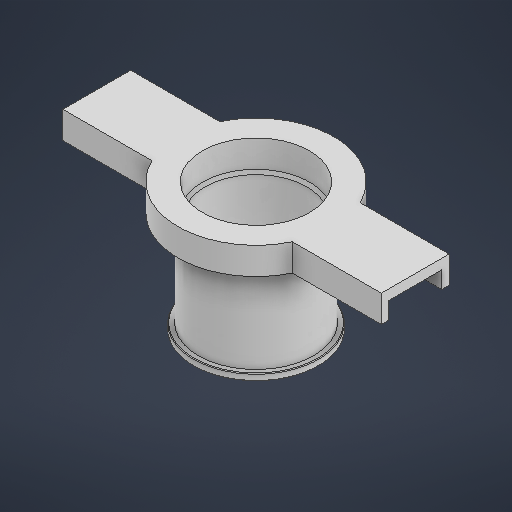
# Autodesk Inventor part: Cylinder  Segment - 11
Saved by Autodesk Inventor 2025 (Build 290162000, 162)
## iProperties
Created: 2024-04-11
Part Number: Cylinder  Segment - 11
Material: Generic
Document SubType Name: Modeling
Designer: Thienan Hoang
Density: 1 g/cm^3
Appearance: Default
Author: Thienan Hoang
Autodesk Inventor part; units mm, degrees
ref_plane "YZ Plane" through (0, 0, 0) normal (1, 0, 0) x (0, 1, 0)
ref_plane "XZ Plane" through (0, 0, 0) normal (0, 1, 0) x (-1, 0, 0)
ref_plane "XY Plane" through (0, 0, 0) normal (0, 0, 1) x (1, 0, 0)
sketch "Sketch1" plane through (0, 0, 0) normal (0, 1, 0) x (-1, 0, 0)
  circle A0 centre (0, 0) radius 46.125
  circle A1 centre (0, 0) radius 42.5
  circle A2 centre (0, 0) radius 37.5
  circle A3 centre (0, 0) radius 9.5
  dimension "Absolute_Diameter" = 92.25
  dimension "Diameter_No_Outer_Lip" = 85
  dimension "Inner_Cylinder_Diameter" = 75
  dimension "Lip_Diameter" = 19
  constraints: 4 centre point, 4 coincident
  measures "Absolute_Diameter" diameter of A0
  measures "Diameter_No_Outer_Lip" diameter of A1
  measures "Inner_Cylinder_Diameter" diameter of A2
  measures "Lip_Diameter" diameter of A3
extrude "Extrusion1" add sketch "Sketch1" along normal blind 5 contours A0
extrude "Extrusion2" add sketch "Sketch1" along normal blind 75 contours A1
sketch "Sketch2" plane through (0, 75, 0) normal (0, 1, 0) x (1, 0, 0)
  circle A0 centre (0, 0) radius 42.5
  circle A1 centre (0, 0) radius 50
  dimension "Lip_Diameter_Out" = 85
  dimension "Inner_Lip_Diameter" = 100
  constraints: 2 centre point, 1 coincident
  measures "Lip_Diameter_Out" diameter of A0
  measures "Inner_Lip_Diameter" diameter of A1
extrude "Extrusion7" [suppressed]
chamfer "Chamfer1" distance 0.5 angle 45 1 edges at (42.5, 75, 0)
chamfer "Chamfer2" distance 0.5 angle 45 3 edges at (46.125, 5, 0) (46.125, 0, 0) (37.5, 0, 0)
sketch "Sketch3" plane through (0, 5, 0) normal (0, 1, 0) x (1, 0, 0)
  circle A0 centre (0, 0) radius 127.5
  circle A1 centre (-127.5, 0) radius 2.5
  circle A2 centre (-103.1497, -74.9426) radius 2.5
  circle A3 centre (-39.3997, -121.2597) radius 2.5
  circle A4 centre (39.3997, -121.2597) radius 2.5
  circle A5 centre (103.1497, -74.9426) radius 2.5
  circle A6 centre (127.5, 0) radius 2.5
  circle A7 centre (103.1497, 74.9426) radius 2.5
  circle A8 centre (39.3997, 121.2597) radius 2.5
  circle A9 centre (-39.3997, 121.2597) radius 2.5
  circle A10 centre (-103.1497, 74.9426) radius 2.5
  dimension "d27" = 255
  dimension "d28" = 5
  dimension "d31" = 360
  constraints: 10 centre point, 1 coincident, 1 horizontal alignment, 23 other
  measures "d28" diameter of A1
extrude "Extrusion8" [suppressed]
chamfer "Chamfer3" distance 2 angle 45 1 edges at (37.5, 75, 0)
sketch "Sketch5" plane through (0, 75, 0) normal (0, 1, 0) x (1, 0, 0)
  circle A0 centre (0, 0) radius 39.5
  circle A1 centre (0, 0) radius 38 projected
  line L0 (117.5, 25) -> (117.5, -25)
  line L1 (-117.5, -25) -> (-117.5, 25)
  line L2 (-117.5, 25) -> (-51.7808, 25)
  line L3 (51.7808, 25) -> (117.5, 25)
  line L4 (117.5, -25) -> (51.7808, -25)
  line L5 (-51.7808, -25) -> (-117.5, -25)
  arc A2 (-51.7808, -25) -> (51.7808, -25) centre (0, 0) ccw
  arc A3 (51.7808, 25) -> (-51.7808, 25) centre (0, 0) ccw
  dimension "d54" = 50
  dimension "d55" = 235
  constraints: 12 end point, 5 parallel, 4 point on circle, 3 centre point, 2 coincident, 2 horizontal, 2 perpendicular
  measures "d54" distance of L0.start L0.end
  measures "d55" distance between parallel lines of L0 L1
extrude "Extrusion9" add sketch "Sketch5" along normal blind 20 contours L0 L4 A2 L5 L1 L2 A3 L3
sketch "Sketch6" plane through (0, 75, 0) normal (0, -1, 0) x (1, 0, 0)
  line L0 (117.25, -22) -> (-117.25, -22)
  line L1 (-117.25, -22) -> (-117.25, 22)
  line L2 (-117.25, 22) -> (117.25, 22)
  line L3 (117.25, 22) -> (117.25, -22)
  line L4 (117.25, -22) -> (-117.25, 22) construction
  line L5 (-117.25, -22) -> (117.25, 22) construction
  line L6 (145.5, -19.625) -> (92, -19.625)
  line L7 (89, -16.625) -> (89, 16.625)
  line L8 (92, 19.625) -> (145.5, 19.625)
  line L9 (145.5, 19.625) -> (145.5, -19.625)
  line L10 (145.5, -19.625) -> (89, 19.625) construction
  line L11 (89, -19.625) -> (145.5, 19.625) construction
  line L12 (-92, -19.625) -> (-145.5, -19.625)
  line L13 (-145.5, -19.625) -> (-145.5, 19.625)
  line L14 (-145.5, 19.625) -> (-92, 19.625)
  line L15 (-89, 16.625) -> (-89, -16.625)
  line L16 (-89, -19.625) -> (-145.5, 19.625) construction
  line L17 (-145.5, -19.625) -> (-89, 19.625) construction
  arc A0 (-92, -19.625) -> (-89, -16.625) centre (-92, -16.625) ccw
  arc A1 (-89, 16.625) -> (-92, 19.625) centre (-92, 16.625) ccw
  arc A2 (89, -16.625) -> (92, -19.625) centre (92, -16.625) ccw
  arc A3 (92, 19.625) -> (89, 16.625) centre (92, 16.625) ccw
  point P0 (0, 0)
  point P1 (117.25, 0)
  point P2 (-117.25, 0)
  dimension "d58" = 234.5
  dimension "d59" = 44
  dimension "d60" = 56.5
  dimension "d61" = 39.25
  dimension "d62" = 56.5
  dimension "d63" = 39.25
  dimension "d64" = 3
  constraints: 36 end point, 8 midpoint, 8 point on circle, 8 point on line, 8 tangent, 6 parallel, 4 centre point, 3 equal radius, 3 horizontal, 3 perpendicular
  measures "d58" distance of L1.end L2.end
  measures "d59" distance of L0.end L1.end
  measures "d60" distance of L10.end L8.end
  measures "d61" distance of L11.start L10.end
  measures "d62" distance of L13.end L17.end
  measures "d63" distance of L12.end L13.end
  measures "d64" radius of A0
extrude "Extrusion10" cut sketch "Sketch6" against normal blind 12.575 contours L6 A2 L7 A3 L8 L3 | L3 L8 L9 L6 | L12 L13 L14 L1 | L1 L14 A1 L15 A0 L12
body "Solid1"
